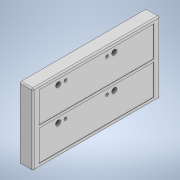
# Autodesk Inventor part: Dual_Backplate
Saved by Autodesk Inventor 2022 (Build 260153000, 153)
## iProperties
Created: 2022-03-29
Part Number: Dual_Backplate
Material: Generic
Document SubType Name: Modeling
Designer: thoms
Density: 1 g/cm^3
Appearance: Default
Author: thoms
Autodesk Inventor part; units mm, degrees
ref_plane "YZ Plane" through (0, 0, 0) normal (1, 0, 0) x (0, 1, 0)
ref_plane "XZ Plane" through (0, 0, 0) normal (0, 1, 0) x (-1, 0, 0)
ref_plane "XY Plane" through (0, 0, 0) normal (0, 0, 1) x (1, 0, 0)
sketch "Sketch1" plane through (0, 0, 0) normal (1, 0, 0) x (0, 1, 0)
  line L0 (14, 25) -> (-14, 25)
  line L1 (-14, 25) -> (-14, -25)
  line L2 (-14, -25) -> (14, -25)
  line L3 (14, -25) -> (14, 25)
  point P0 (0, 0)
  dimension "d0" = 50
  dimension "d1" = 25
  dimension "d2" = 28
  dimension "d3" = 14
  constraints: 8 end point, 2 parallel, 1 horizontal, 1 perpendicular
  measures "d0" distance of L2.end L0.start
  measures "d1" distance from line of point (0, 0) L0
  measures "d2" distance of L0.start L0.end
  measures "d3" distance from line of point (0, 0) L3
extrude "Extrusion1" add sketch "Sketch1" against normal blind 5
sketch "Sketch2" plane through (0, 0, 0) normal (1, 0, 0) x (0, 0, -1)
  circle A0 centre (-12.1, 10.5) radius 0.55
  circle A1 centre (-14.95, 10.5) radius 1
  circle A2 centre (4.25, 10.5) radius 0.55
  circle A3 centre (7.1, 10.5) radius 1
  line L0 (25, -14) -> (25, 14) projected
  line L1 (-25, 14) -> (-25, -14) projected
  line L2 (-14.95, 10.5) -> (7.1, 10.5) construction
  line L3 (-25, -14) -> (25, -14) projected
  line L4 (25, 14) -> (-25, 14) projected
  line L5 (-8.2421, 4) -> (2.4524, 4) construction
  circle A4 centre (-12.1, -2.5) radius 0.55
  circle A5 centre (-14.95, -2.5) radius 1
  circle A6 centre (4.25, -2.5) radius 0.55
  circle A7 centre (7.1, -2.5) radius 1
  line L6 (-14.95, -2.5) -> (7.1, -2.5) construction
  point P0 (0, 0)
  dimension "d6" = 2
  dimension "d7" = 2
  dimension "d8" = 1.1
  dimension "d9" = 1.1
  dimension "d11" = 2.85
  dimension "d13" = 2.85
  dimension "d14" = 10.05
  dimension "d19" = 16.35
  dimension "d20" = 3.5
  dimension "d28" = 10
  constraints: 8 centre point, 6 end point, 4 symmetric about line, 2 horizontal, 4 other
  measures "d6" diameter of A1
  measures "d7" diameter of A3
  measures "d8" diameter of A0
  measures "d9" diameter of A2
  measures "d11" distance of A0.centre L2.start
  measures "d13" distance of L2.end A2.centre
  measures "d14" distance from line of L1 L2.start
  measures "d19" distance of A2.centre A0.centre
  measures "d20" distance between parallel lines of L4 L2
  measures "d28" distance between parallel lines of L4 L5
extrude "Extrusion2" cut sketch "Sketch2" against normal up to surface (5 mm away) contours A0 | A1 | A2 | A3 | A4 | A5 | A6 | A7
fillet "Fillet1" radius 0.5 8 edges at (0, 0, 25) (0, 14, 0) (0, 0, -25) (0, -14, 0) (-2.5, 14, 25) (-2.5, -14, 25) (-2.5, 14, -25) (-2.5, -14, -25)
sketch "Sketch3" plane through (0, 0, 0) normal (1, 0, 0) x (0, 0, -1)
  line L0 (-22.5, 12.5) -> (22.6, 12.5)
  line L1 (22.6, 12.5) -> (22.6, 0.5)
  line L2 (22.6, 0.5) -> (-22.5, 0.5)
  line L3 (-22.5, 0.5) -> (-22.5, 12.5)
  circle A0 centre (-14.95, 10.5) radius 1 projected
  line L4 (0, 0) -> (3.2775, 0) construction
  line L5 (-22.5, -12.5) -> (22.6, -12.5)
  line L6 (22.6, -12.5) -> (22.6, -0.5)
  line L7 (22.6, -0.5) -> (-22.5, -0.5)
  line L8 (-22.5, -0.5) -> (-22.5, -12.5)
  dimension "d21" = 45.1
  dimension "d22" = 7.55
  dimension "d23" = 10
  dimension "d24" = 2
  constraints: 18 end point, 4 symmetric about line, 2 horizontal, 2 parallel, 1 perpendicular
  measures "d21" distance of L0.start L0.end
  measures "d22" distance from line of A0.centre L3
  measures "d23" distance from line of A0.centre L2
  measures "d24" distance from line of A0.centre L0
extrude "Extrusion3" cut sketch "Sketch3" against normal blind 0.1
body "Solid1"
